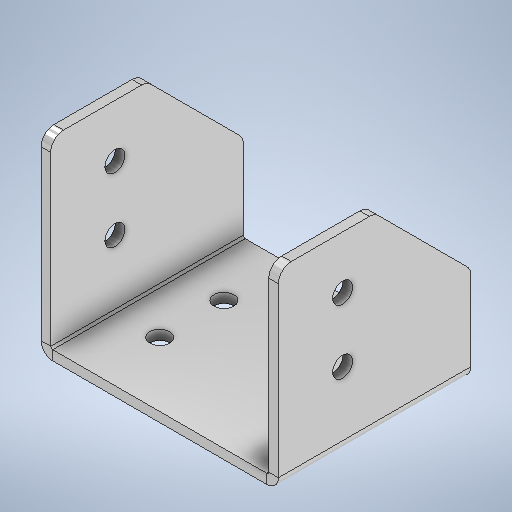
# Autodesk Inventor part: Head1
Saved by Autodesk Inventor 2026.1 (Build 301233000, 233)
## iProperties
Created: 2025-08-16
Part Number: Head1
Material: Aluminum 6061-AHC
Document SubType Name: Sheet Metal
Designer: chris
Density: 2.7 g/cm^3
Sheet Metal Rule: Default_mm
Appearance: Aluminum - Dark
Flat Pattern Width: 3 cm
Flat Pattern Length: 9.15586 cm
Flat Pattern Area: 27.4676 cm^2
Sheet Metal Width: 30.000 mm
Sheet Metal Length: 91.559 mm
Sheet Metal Area: 2746.757 mm^2
Author: chris
Autodesk Inventor part; units mm, degrees
note: some values were not read from the file. Chosen so that the rebuilt part matches the saved one: flange form of "Plate2".
ref_plane "YZ Plane" through (0, 0, 0) normal (1, 0, 0) x (0, 1, 0)
ref_plane "XZ Plane" through (0, 0, 0) normal (0, 1, 0) x (-1, 0, 0)
ref_plane "XY Plane" through (0, 0, 0) normal (0, 0, 1) x (1, 0, 0)
sketch "Sketch1" plane through (0, 0, 0) normal (0, 1, 0) x (-1, 0, 0)
  line L0 (18.5, 15) -> (-18.5, 15)
  line L1 (-18.5, 15) -> (-18.5, -15)
  line L2 (-18.5, -15) -> (18.5, -15)
  line L3 (18.5, -15) -> (18.5, 15)
  line L4 (18.5, 15) -> (-18.5, -15) construction
  line L5 (-18.5, 15) -> (18.5, -15) construction
  circle A0 centre (10, 5) radius 1.55
  circle A1 centre (10, -5) radius 1.55
  circle A2 centre (-10, 5) radius 1.55
  circle A3 centre (-10, -5) radius 1.55
  point P0 (0, 0)
  dimension "d0" = 37
  dimension "d1" = 30
  dimension "d2" = 3.1
  dimension "d3" = 3.1
  dimension "d4" = 3.1
  dimension "d5" = 3.1
  dimension "d6" = 20
  dimension "d7" = 20
  dimension "d8" = 10
  dimension "d10" = 10
  dimension "d11" = 0
  dimension "d12" = 0
  dimension "d13" = 10
  dimension "d14" = 8.5
  measures "d0" distance of L0.start L0.end
  measures "d1" distance of L0.end L1.end
  measures "d2" diameter of A0
  measures "d3" diameter of A1
  measures "d4" diameter of A2
  measures "d5" diameter of A3
  measures "d6" distance of A0.centre A2.centre
  measures "d7" distance of A1.centre A3.centre
  measures "d8" distance of A3.centre A2.centre
  measures "d10" distance of A1.centre A0.centre
  measures "d11" horizontal distance of A3.centre A2.centre
  measures "d12" vertical distance of A0.centre A2.centre
  measures "d13" distance from line of L0 A2.centre
  measures "d14" distance from line of L1 A2.centre
extrude "Plate1" add sketch "Sketch1" along normal blind 1.5
sketch "Sketch2" plane through (17, 0, -15) normal (1, 0, 0) x (0, 1, 0)
  line L0 (0, 30) -> (0, 0)
  line L1 (0, 0) -> (30, 0)
  line L2 (30, 0) -> (30, 30)
  line L3 (30, 30) -> (0, 30)
  constraints: 6 end point, 1 horizontal, 1 perpendicular, 1 vertical
edge flange "Flange1" height 30 angle 90 thickness 1.5 bend radius 0.31 thickness toward (1, 0, 0) relief tear relief width 1.5 relief depth 0.75 corner gap 0.31 corner form 0 edges at (18.5, 1.5, 0) (-18.5, 1.5, 0) wall of the first edge with corners at (17, 0, 15) (17, 0, -15) (17, 30, -15) (17, 30, 15)
bend "Bend1"
corner "Corner1"
sketch "Sketch3" plane through (18.5, 30, 15) normal (1, 0, 0) x (0, 0, -1)
  circle A0 centre (10, -8.19) radius 1.55
  circle A1 centre (10, -18.19) radius 1.55
  line L0 (0, -28.19) -> (0, 0) projected
  line L1 (0, -28.19) -> (30, -28.19) projected
  point P0 (15, -30)
  dimension "d26" = 3.1
  dimension "d27" = 3.1
  dimension "d28" = 10
  dimension "d29" = 10
  dimension "d30" = 10
  dimension "d31" = 10
  constraints: 2 centre point
  measures "d26" diameter of A0
  measures "d27" diameter of A1
  measures "d28" distance from line of L0 A1.centre
  measures "d29" distance from line of L0 A0.centre
  measures "d30" distance of A1.centre A0.centre
  measures "d31" distance from line of L1 A1.centre
extrude "Cut1" cut sketch "Sketch3" against normal through all
sketch "Sketch5" plane through (18.5, 30, 15) normal (1, 0, 0) x (0, 0, -1)
  line L0 (15, 0) -> (30, -15)
  line L1 (30, -15) -> (30, 0)
  line L2 (30, 0) -> (15, 0)
  line L3 (30, 0) -> (30, -28.19) projected
  line L4 (0, 0) -> (30, 0) projected
  point P0 (15, -30)
  dimension "d36" = 15
  dimension "d37" = 15
  constraints: 7 end point, 2 collinear, 1 perpendicular, 1 vertical
  measures "d36" distance of L1.end L0.start
  measures "d37" distance of L0.end L1.end
extrude "Cut2" cut sketch "Sketch5" against normal through all
fillet "Fillet1" radius 2 6 edges at (17.75, 30, 15) (17.75, 30, 0) (17.75, 15, -15) (-17.75, 30, 15) (-17.75, 30, 0) (-17.75, 15, -15)
equation "\"d7\" = d6"
equation "\"d10\" = d8"
equation "\"d32\" = Thickness"
equation "\"d38\" = Thickness"
equation "\"d15\" = Thickness"
equation "\"d16\" = BendReliefWidth"
equation "\"d17\" = BendReliefDepth"
equation "\"d18\" = MinimumRemnant"
equation "\"d19\" = TransitionRadius"
equation "\"d22\" = BendRadius"
equation "\"d23\" = CornerReliefSize"
equation "\"d24\" = GapSize"
equation "\"d25\" = JacobiRadiusSize"
equation "\"BendReliefWidth\" = Thickness"
equation "\"BendReliefDepth\" = 0.5 * Thickness"
equation "\"CornerReliefSize\" = 4 * Thickness"
equation "\"MinimumRemnant\" = 2 * Thickness"
equation "\"TransitionRadius\" = BendRadius"
equation "\"JacobiRadiusSize\" = BendRadius"
equation "\"GapSize\" = Thickness"
equation "\"Thickness\" = 1.5"
equation "\"BendRadius\" = 0.31"
body "Solid1"
